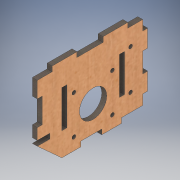
# Autodesk Inventor part: stepperMount
Saved by Autodesk Inventor 2019 (Build 230136000, 136)
## iProperties
Created: 2020-12-06
Part Number: stepperMount
Material: Дерево (береза)
Document SubType Name: Modeling
Designer: Professional
Density: 0.55 g/cm^3
Appearance: Береза — натуральный — полированный
Author: Professional
Autodesk Inventor part; units mm, degrees
ref_plane "YZ Plane" through (0, 0, 0) normal (1, 0, 0) x (0, 1, 0)
ref_plane "XZ Plane" through (0, 0, 0) normal (0, 1, 0) x (-1, 0, 0)
ref_plane "XY Plane" through (0, 0, 0) normal (0, 0, 1) x (1, 0, 0)
sketch "Эскиз1" plane through (0, 0, 0) normal (1, 0, 0) x (0, 1, 0)
  line L0 (0, 0) -> (8, 0)
  line L1 (8, 0) -> (8, -4)
  line L2 (8, -4) -> (22, -4)
  line L3 (22, -4) -> (22, 0)
  line L4 (22, 0) -> (38, 0)
  line L5 (38, 0) -> (38, -4)
  line L6 (38, -4) -> (52, -4)
  line L7 (52, -4) -> (52, 0)
  line L8 (52, 0) -> (60, 0)
  line L9 (60, 0) -> (60, 12)
  line L10 (60, 12) -> (64, 12)
  line L11 (64, 12) -> (64, 32)
  line L12 (64, 32) -> (60, 32)
  line L13 (60, 32) -> (60, 53)
  line L14 (60, 53) -> (64, 53)
  line L15 (64, 53) -> (64, 73)
  line L16 (64, 73) -> (60, 73)
  line L17 (60, 73) -> (60, 85)
  line L18 (-4, 65.2) -> (-4, 50)
  line L19 (-4, 50) -> (0, 50)
  line L20 (0, 50) -> (0, 33)
  line L21 (0, 33) -> (-4, 33)
  line L22 (-4, 33) -> (-4, 17)
  line L23 (-4, 17) -> (0, 17)
  line L24 (0, 17) -> (0, 0)
  line L25 (0, 61.2) -> (42.4, 61.2) construction
  line L26 (42.4, 61.2) -> (42.4, 18.8) construction
  line L27 (42.4, 18.8) -> (0, 18.8) construction
  line L28 (0, 18.8) -> (0, 61.2) construction
  line L29 (42.4, 61.2) -> (0, 18.8) construction
  line L30 (0, 61.2) -> (42.4, 18.8) construction
  circle A0 centre (21.2, 40) radius 11
  circle A1 centre (36.7, 55.5) radius 1.5
  circle A2 centre (36.7, 24.5) radius 1.5
  circle A3 centre (5.7, 24.5) radius 1.5
  circle A4 centre (5.7, 55.5) radius 1.5
  line L31 (-4, 65.2) -> (14, 85)
  line L32 (27, 85) -> (27, 81)
  line L33 (27, 81) -> (47, 81)
  line L34 (47, 81) -> (47, 85)
  line L35 (47, 85) -> (60, 85)
  line L36 (15, 14.8) -> (45, 14.8)
  line L37 (45, 14.8) -> (45, 18.8)
  line L38 (45, 18.8) -> (15, 18.8)
  line L39 (15, 18.8) -> (15, 14.8)
  line L40 (15, 61.2) -> (45, 61.2)
  line L41 (45, 61.2) -> (45, 65.2)
  line L42 (45, 65.2) -> (15, 65.2)
  line L43 (15, 65.2) -> (15, 61.2)
  line L44 (14, 85) -> (14, 75)
  line L45 (14, 75) -> (18, 75)
  line L46 (18, 75) -> (18, 85)
  line L47 (18, 85) -> (27, 85)
  point P0 (21.2, 40)
  point P1 (30, 14.8)
  point P2 (30, 0)
  dimension "d0" = 4
  dimension "d1" = 8
  dimension "d2" = 14
  dimension "d3" = 16
  dimension "d4" = 14
  dimension "d5" = 8
  dimension "d6" = 17
  dimension "d7" = 16
  dimension "d8" = 17
  dimension "d9" = 15.2
  dimension "d11" = 12
  dimension "d12" = 20
  dimension "d13" = 20
  dimension "d16" = 21
  dimension "d22" = 42.4
  dimension "d23" = 31
  dimension "d24" = 40
  dimension "d25" = 22
  dimension "d26" = 3
  dimension "d31" = 85
  dimension "d32" = 12
  dimension "d33" = 20
  dimension "d36" = 30
  dimension "d37" = 10
  dimension "d38" = 13
  dimension "d40" = 13
  constraints: 96 end point, 24 perpendicular, 17 point on line, 10 equal length, 9 horizontal, 7 parallel, 5 centre point, 5 midpoint, 5 vertical alignment, 4 coincident, 4 horizontal alignment, 3 equal radius, 2 vertical
  measures "d0" distance of L0.end L1.end
  measures "d1" distance of L0.start L0.end
  measures "d2" distance of L1.end L2.end
  measures "d3" distance between parallel lines of L3 L5
  measures "d4" distance of L5.end L6.end
  measures "d5" distance between parallel lines of L9 L7
  measures "d6" distance between parallel lines of L0 L23
  measures "d7" distance of L21.end L22.end
  measures "d8" distance of L19.end L20.end
  measures "d9" distance of L18.start L18.end
  measures "d11" distance between parallel lines of L8 L10
  measures "d12" distance of L10.end L11.end
  measures "d13" distance of L14.end L15.end
  measures "d16" distance between parallel lines of L12 L14
  measures "d22" distance between parallel lines of L27 L25
  measures "d23" distance of point (36.7, 24.5) point (36.7, 55.5)
  measures "d24" distance from line of point (21.2, 40) L4
  measures "d25" diameter of A0
  measures "d26" diameter of A1
  measures "d31" distance between parallel lines of L8 L35
  measures "d32" distance between parallel lines of L35 L16
  measures "d33" distance between parallel lines of L34 L32
  measures "d36" distance between parallel lines of L39 L37
  measures "d37" distance of L45.end L46.end
  measures "d38" distance between parallel lines of L34 L17
  measures "d40" distance between parallel lines of L32 L44
extrude "Выдавливание1" add sketch "Эскиз1" along normal blind 4
sketch "Эскиз4" plane through (4, 0, 0) normal (1, 0, 0) x (0, 0, -1)
  line L0 (0, 0) -> (0, 8) projected
  line L1 (-14.8, 45) -> (-14.8, 15) projected
  line L2 (-17, 0) -> (0, 0) projected
  line L3 (0, 60) -> (-12, 60) projected
  point P0 (-9.8, 14)
  point P1 (-9.8, 46)
  dimension "d51" = 5
  dimension "d52" = 14
  dimension "d53" = 14
  constraints: 1 vertical alignment
  measures "d51" distance from line of L1 point (-9.8, 14)
  measures "d52" distance from line of L2 point (-9.8, 14)
  measures "d53" distance from line of L3 point (-9.8, 46)
hole "Отверстие1" at (4, 14, 9.8) at (4, 46, 9.8) direction (-1, 0, 0) diameter 3 end through all
